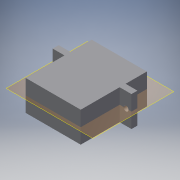
# Autodesk Inventor part: servo
Saved by Autodesk Inventor 2018 (Build 220112000, 112)
## iProperties
Created: 2017-12-09
Part Number: servo
Material: Generic
Document SubType Name: Modeling
Designer: ragna
Density: 1 g/cm^3
Appearance: Default
Author: ragna
Autodesk Inventor part; units mm, degrees
ref_plane "YZ Plane" through (0, 0, 0) normal (1, 0, 0) x (0, 1, 0)
sketch "Sketch1" plane through (0, 0, 0) normal (0, 1, 0) x (-1, 0, 0)
  line L0 (0, 0) -> (22.6, 0)
  line L1 (22.6, 0) -> (22.6, -12.4)
  line L2 (22.6, -12.4) -> (0, -12.4)
  line L3 (0, -12.4) -> (0, 0)
  dimension "d0" = 22.6
  dimension "d1" = 12.4
  constraints: 8 end point, 2 parallel, 1 horizontal, 1 perpendicular
  measures "d0" distance of L1.end L2.end
  measures "d1" distance of L0.end L1.end
extrude "Extrusion1" add sketch "Sketch1" along normal blind 27.1
sketch "Sketch2" plane through (0, 27.1, 0) normal (0, 1, 0) x (1, 0, 0)
  circle A0 centre (-16.6, 6.2) radius 2.4
  line L0 (-22.6, 12.4) -> (-22.6, 0) projected
  line L1 (-22.6, 0) -> (0, 0) projected
  line L2 (0, 12.4) -> (-22.6, 12.4) projected
  dimension "d4" = 4.8
  dimension "d5" = 6
  dimension "d6" = 6.2
  dimension "d7" = 6.2
  constraints: 1 centre point
  measures "d4" diameter of A0
  measures "d5" distance from line of L0 A0.centre
  measures "d6" distance from line of L1 A0.centre
  measures "d7" distance from line of L2 A0.centre
extrude "Extrusion2" add sketch "Sketch2" along normal blind 3.1
sketch "Sketch3" plane through (0, 0, 0) normal (1, 0, 0) x (0, 0, -1)
  line L0 (0, 0) -> (0, 27.1) projected
  line L1 (12.4, 0) -> (12.4, 27.1) projected
  line L2 (0, 18.4) -> (12.4, 18.4)
  line L3 (12.4, 18.4) -> (12.4, 15.95)
  line L4 (12.4, 15.95) -> (0, 15.95)
  line L5 (0, 15.95) -> (0, 18.4)
  line L6 (0, 27.1) -> (12.4, 27.1) projected
  dimension "d10" = 2.45
  dimension "d11" = 8.7
  constraints: 8 end point, 2 parallel, 2 point on line, 1 horizontal, 1 perpendicular
  measures "d10" distance of L2.end L3.end
  measures "d11" distance between parallel lines of L2 L6
extrude "Extrusion3" add sketch "Sketch3" along normal blind 4.85 contours L0 L2 L1 L4
ref_plane "Work Plane1" through (-11.3, 27.1, 0) normal (1, 0, 0) x (0, 0, -1)
mirror "Mirror1" about plane through (-11.3, 27.1, 0) normal (1, 0, 0) of "Extrusion3"
sketch "Sketch4" plane through (0, 18.4, 0) normal (0, 1, 0) x (1, 0, 0)
  circle A0 centre (2.6, 6.2) radius 1.05
  line L0 (-11.3, 14.88) -> (-11.3, -2.48) projected
  line L1 (0, 12.4) -> (4.85, 12.4) projected
  line L2 (0, 0) -> (4.85, 0) projected
  dimension "d14" = 2.1
  dimension "d15" = 13.9
  dimension "d16" = 6.2
  dimension "d17" = 6.2
  constraints: 1 centre point
  measures "d14" diameter of A0
  measures "d15" distance from line of L0 A0.centre
  measures "d16" distance from line of L1 A0.centre
  measures "d17" distance from line of L2 A0.centre
extrude "Extrusion4" cut sketch "Sketch4" against normal through all
mirror "Mirror2" about plane through (-11.3, 27.1, 0) normal (1, 0, 0) of "Extrusion4"
ref_plane "Work Plane3" through (-16.6, 27.1, -6.2) normal (-1, 0, 0) x (0, 0, 1)
ref_plane "Work Plane4" through (-22.6, 0, -6.2) normal (0, 0, 1) x (1, 0, 0)
ref_plane "Work Plane2" through (-11.3, 27.1, 0) normal (1, 0, 0) x (0, 0, -1)
equation "\"d7\" = d6"
equation "\"d17\" = d16"
body "Solid1"
